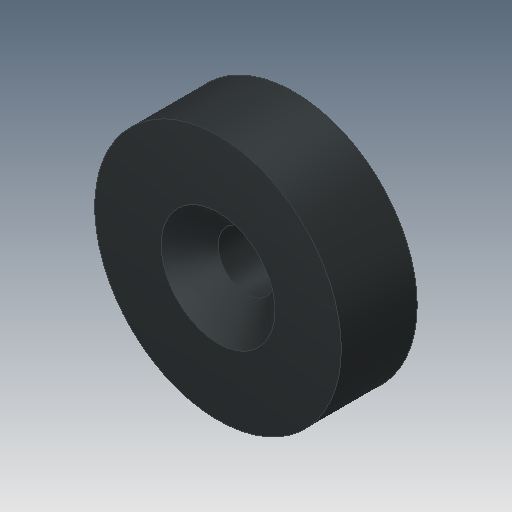
# Autodesk Inventor part: magnetic_annular_body_v2
Saved by Autodesk Inventor 2021.4 (Build 254397000, 397)
## iProperties
Created: 2020-05-18
Part Number: magnetic_annular_body_v2
Material: Eisen, duktil
Document SubType Name: Modeling
Designer: Alex
Mass: 3.4929 g
Surface Area: 4.47036 cm^2
Volume: 0.488518 cm^3
Density: 7.15 g/cm^3
Appearance: Eisen - Grau
Author: Alex
Autodesk Inventor part; units mm, degrees
ref_plane "YZ Plane" through (0, 0, 0) normal (1, 0, 0) x (0, 1, 0)
ref_plane "XY Plane" through (0, 0, 0) normal (0, 0, 1) x (1, 0, 0)
sketch "Skizze1" plane through (0, 0, 0) normal (0, 0, 1) x (1, 0, 0)
  circle A0 centre (0, 0) radius 1.5
  circle A1 centre (0, 0) radius 6.5
  dimension "d0" = 3
  dimension "d1" = 13
  constraints: 2 centre point, 2 coincident
  measures "d0" diameter of A0
  measures "d1" diameter of A1
extrude "Grundkörper" add sketch "Skizze1" along normal blind 4
ref_plane "Work Plane1" through (0, 0, 0) normal (0, 1, 0) x (0, 0, 1)
sketch "Sketch2" plane through (0, 0, 0) normal (0, 1, 0) x (0, 0, 1)
  line L0 (4, -3) -> (1, 0)
  line L1 (1, 0) -> (4, 3)
  line L2 (4, 3) -> (4, -3)
  line L3 (1, 0) -> (4, 0)
  line L4 (-0.8, 0) -> (4.8, 0) projected
  line L5 (4, -6.5) -> (4, 6.5) construction
  point P0 (0, 0)
  dimension "d14" = 90
  dimension "d15" = 6
  constraints: 8 end point, 2 collinear, 1 midpoint, 1 perpendicular, 1 vertical
  measures "d14" angle of L1 L0
  measures "d15" distance of L1.end L0.start
revolve "Revolution1" cut sketch "Sketch2" angle 360 about axis through (0, 0, 0) along (0, 0, 1) contours L0 L3 L2
